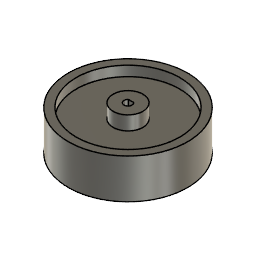
Wheel (Autodesk Fusion 360 design; units mm, degrees)
part number: 2026-04-02-18-33-10-450
Autodesk Fusion 360 part; units mm, degrees
sketch "Sketch1" plane through (0, 0, 0) normal (0, 0, 1) x (1, 0, 0)
  circle A0 centre (0, 0) radius 30
  circle A1 centre (0, 0) radius 2.05
  line L0 (0, -2.05) -> (0, 1.55) construction
  line L1 (0, 1.55) -> (1.3416, 1.55)
  line L2 (0, 1.55) -> (-1.3416, 1.55)
  dimension "d1" = 60
  dimension "d2" = 4.1
  dimension "d6" = 3.6
  constraint coincident A0.centre A1.centre
  constraint concentric A0 A1
  constraint coincident A1 L0.start
  constraint vertical L0
  constraint coincident A1 L1.end
  constraint perpendicular L0 L1
  constraint coincident A1 L2.end
  constraint perpendicular L0 L2
  measures "d1" diameter of A0
  measures "d2" diameter of A1
  measures "d6" distance of L0.start L0.end
extrude "Extrude1" add sketch "Sketch1" along normal blind 20 contours A0 | A1 L1 L2 picked at (-0.0972, 1.8764)
sketch "Sketch2" plane through (0, 0, 20) normal (0, 0, 1) x (-1, 0, 0)
  line L0 (1.3416, -1.55) -> (-1.3416, -1.55)
  arc A0 (1.3416, -1.55) -> (-1.3416, -1.55) centre (0, 0) ccw
  circle A1 centre (0, 0) radius 30
  circle A2 centre (0, 0) radius 7.5
  circle A3 centre (0, 0) radius 26
  dimension "d7" = 15
  dimension "d8" = 52
  constraint concentric A0 A2
  constraint concentric A0 A3
  measures "d7" diameter of A2
  measures "d8" diameter of A3
extrude "Extrude2" cut sketch "Sketch2" against normal blind 5 contours A3
extrude "Extrude3" add sketch "Sketch2" along normal blind 2 contours A2
sketch "Sketch3" plane through (0, 0, 0) normal (0, 0, 1) x (1, 0, 0)
  circle A0 centre (0, 0) radius 26
  dimension "d14" = 52
  measures "d14" diameter of A0
extrude "Extrude4" cut sketch "Sketch1" sketch "Sketch3" along normal blind 5 contours A1 L1 L2 | A1 L1 L2 of sketch 2
